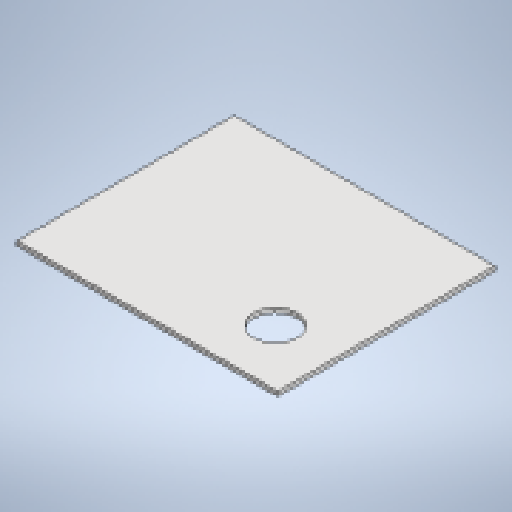
# Autodesk Inventor part: PNS-071 stretch ring
Saved by Autodesk Inventor 2025 (Build 290162010, 162A)
## iProperties
Created: 2025-03-26
Part Number: PNS-071 stretch ring
Material: Stainless Steel
Description: DIE16(5)|\ 90°|corrY -___°|X_____|bom___
Document SubType Name: Sheet Metal
Designer: admin
Stock Number: МОО 305 шпангоут борт
Mass: 1762.25 g
Surface Area: 2283.33 cm^2
Volume: 220.281 cm^3
Density: 8 g/cm^3
Sheet Metal Rule: AISI304 2mm Die16
Sheet Metal Width: 0.000 mm
Sheet Metal Length: 0.000 mm
Sheet Metal Area: 0.000 mm^2
Appearance: Default
Author: admin
Autodesk Inventor part; units mm, degrees
ref_plane "YZ Plane" through (0, 0, 0) normal (1, 0, 0) x (0, 1, 0)
ref_plane "XZ Plane" through (0, 0, 0) normal (0, 1, 0) x (-1, 0, 0)
ref_plane "XY Plane" through (0, 0, 0) normal (0, 0, 1) x (1, 0, 0)
sketch "Sketch1" plane through (0, 0, 0) normal (0, 0, 1) x (1, 0, 0)
  line L0 (-60, -50) -> (60, -50)
  line L1 (60, -50) -> (60, 50)
  line L2 (60, 50) -> (-60, 50)
  line L3 (-60, 50) -> (-60, -50)
  line L4 (-60, -50) -> (60, 50) construction
  line L5 (60, -50) -> (-60, 50) construction
  circle A0 centre (33.1903, -24.2194) radius 10
  point P0 (0, 0)
  dimension "d154" = 120
  dimension "d155" = 100
  dimension "d157" = 20
  measures "d154" distance of L1.end L2.end
  measures "d155" distance of L0.end L1.end
  measures "d157" diameter of A0
extrude "Plate5" add sketch "Sketch1" along normal blind 2
body "Solid3"
